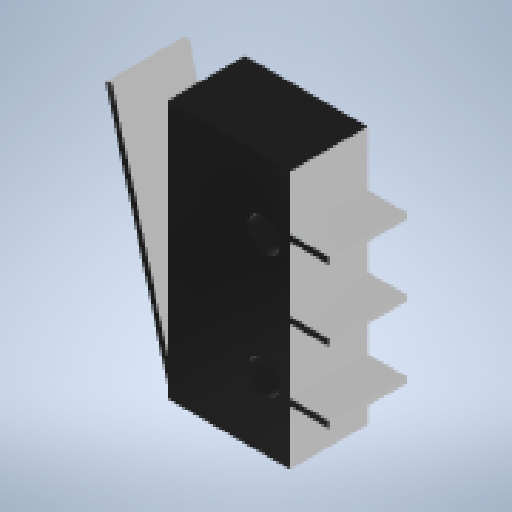
# Autodesk Inventor part: RefSwitch_Basic
Saved by Autodesk Inventor 2023.2 (Build 272271000, 271)
## iProperties
Created: 2022-06-22
Part Number: RefSwitch_Basic
Material: Aluminum 6061
Document SubType Name: Modeling
Designer: Remo
Density: 2.7 g/cm^3
Appearance: Aluminum - Flat
Author: Remo
Autodesk Inventor part; units mm, degrees
ref_plane "YZ Plane" through (0, 0, 0) normal (1, 0, 0) x (0, 1, 0)
ref_plane "XZ Plane" through (0, 0, 0) normal (0, 1, 0) x (-1, 0, 0)
ref_plane "XY Plane" through (0, 0, 0) normal (0, 0, 1) x (1, 0, 0)
sketch "Sketch1" plane through (0, 0, 0) normal (0, 0, 1) x (1, 0, 0)
  line L0 (4.75, -10) -> (-4.75, -10)
  line L1 (-4.75, -10) -> (-4.75, 10)
  line L2 (-4.75, 10) -> (4.75, 10)
  line L3 (4.75, 10) -> (4.75, -10)
  line L4 (4.75, -10) -> (-4.75, 10) construction
  line L5 (-4.75, -10) -> (4.75, 10) construction
  circle A0 centre (2.75, 4.75) radius 1.25
  circle A1 centre (2.75, -4.75) radius 1.25
  line L6 (-4.75, -7.0681) -> (-9.0554, 9)
  line L7 (-9.0554, 9) -> (-9.5384, 8.8706)
  line L8 (-9.5384, 8.8706) -> (-4.75, -9)
  line L9 (7.75, -0.25) -> (4.75, -0.25)
  line L10 (4.75, -0.25) -> (4.75, 0.25)
  line L11 (4.75, 0.25) -> (7.75, 0.25)
  line L12 (7.75, 0.25) -> (7.75, -0.25)
  line L13 (7.75, -0.25) -> (4.75, 0.25) construction
  line L14 (4.75, -0.25) -> (7.75, 0.25) construction
  line L15 (4.75, -5.25) -> (7.75, -5.25)
  line L16 (7.75, -5.25) -> (7.75, -5.75)
  line L17 (7.75, -5.75) -> (4.75, -5.75)
  line L18 (4.75, -5.75) -> (4.75, -5.25)
  line L19 (4.75, -5.25) -> (7.75, -5.75) construction
  line L20 (7.75, -5.25) -> (4.75, -5.75) construction
  line L21 (4.75, 5.75) -> (7.75, 5.75)
  line L22 (7.75, 5.75) -> (7.75, 5.25)
  line L23 (7.75, 5.25) -> (4.75, 5.25)
  line L24 (4.75, 5.25) -> (4.75, 5.75)
  line L25 (4.75, 5.75) -> (7.75, 5.25) construction
  line L26 (7.75, 5.75) -> (4.75, 5.25) construction
  point P0 (0, 0)
  point P1 (6.25, 0)
  point P2 (6.25, -5.5)
  point P3 (6.25, 5.5)
  point P4 (6.25, 0.25)
  dimension "d0" = 20
  dimension "d1" = 9.5
  dimension "d2" = 2.5
  dimension "d3" = 9.5
  dimension "d4" = 4.75
  dimension "d5" = 2
  dimension "d6" = 0.5
  dimension "d7" = 15
  dimension "d8" = 1
  dimension "d9" = 1
  dimension "d12" = 0.5
  dimension "d13" = 3
  dimension "d14" = 5
  dimension "d15" = 5
  constraints: 54 end point, 9 midpoint, 9 parallel, 5 perpendicular, 4 equal length, 4 horizontal, 4 point on line, 2 centre point, 2 vertical alignment, 1 equal radius, 1 horizontal alignment
  measures "d0" distance of L0.end L1.end
  measures "d1" distance of L1.end L2.end
  measures "d2" diameter of A0
  measures "d3" distance of A1.centre A0.centre
  measures "d4" vertical distance of A1.centre point (0, 0)
  measures "d5" distance from line of L3 A0.centre
  measures "d6" distance between parallel lines of L8 L6
  measures "d7" angle of L1 L6
  measures "d8" distance of L0.end L8.end
  measures "d9" distance from line of L2 L6.end
  measures "d12" distance of L11.end L9.start
  measures "d13" distance between parallel lines of L3 L12
  measures "d14" distance from line of L23 point (6.25, 0.25)
  measures "d15" distance between parallel lines of L9 L15
extrude "Extrusion1" add sketch "Sketch1" along normal blind 6
equation "\"d4\" = 0.5 * d3"
equation "\"d9\" = d8"
equation "\"d15\" = d14"
body "Solid1"
